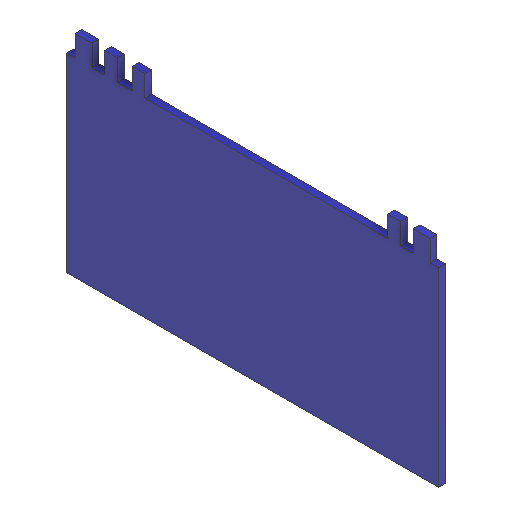
# Autodesk Inventor part: PCB_2
Saved by Autodesk Inventor 2025.2 (Build 292293000, 293)
## iProperties
Created: 2025-03-09
Part Number: PCB_2
Material: Generic
Document SubType Name: Modeling
Designer: ahorat
Density: 1 g/cm^3
Appearance: Default
Author: ahorat
Autodesk Inventor part; units mm, degrees
ref_plane "YZ Plane" through (0, 0, 0) normal (1, 0, 0) x (0, 1, 0)
ref_plane "XZ Plane" through (0, 0, 0) normal (0, 1, 0) x (-1, 0, 0)
ref_plane "XY Plane" through (0, 0, 0) normal (0, 0, 1) x (1, 0, 0)
sketch "Sketch1" plane through (0, 0, 0) normal (0, 0, 1) x (1, 0, 0)
  line L0 (-44, -22.5) -> (44, -22.5)
  line L1 (44, -22.5) -> (44, 22.5)
  line L2 (44, 22.5) -> (-44, 22.5)
  line L3 (-44, 22.5) -> (-44, -22.5)
  line L4 (-44, -22.5) -> (44, 22.5) construction
  line L5 (44, -22.5) -> (-44, 22.5) construction
  line L6 (-42, 22.5) -> (-42, 27.5)
  line L7 (-42, 27.5) -> (-38, 27.5)
  line L8 (-38, 27.5) -> (-38, 22.5)
  line L9 (-35, 22.5) -> (-35, 27.5)
  line L10 (-35, 27.5) -> (-32, 27.5)
  line L11 (-32, 27.5) -> (-32, 22.5)
  line L12 (-28.5, 22.5) -> (-28.5, 27.5)
  line L13 (-28.5, 27.5) -> (-25.5, 27.5)
  line L14 (-25.5, 27.5) -> (-25.5, 22.5)
  line L15 (32, 22.5) -> (32, 27.5)
  line L16 (32, 27.5) -> (35, 27.5)
  line L17 (35, 27.5) -> (35, 22.5)
  line L18 (38, 22.5) -> (38, 27.5)
  line L19 (38, 27.5) -> (42, 27.5)
  line L20 (42, 27.5) -> (42, 22.5)
  point P0 (0, 0)
  point P1 (-28.5, 25)
  point P2 (-40, 27.5)
  dimension "d0" = 45
  dimension "d1" = 88
  dimension "d2" = 4
  dimension "d3" = 3
  dimension "d4" = 3
  dimension "d5" = 3
  dimension "d6" = 4
  dimension "d7" = 2
  dimension "d8" = 3
  dimension "d9" = 3.5
  dimension "d10" = 2
  dimension "d11" = 3
  dimension "d12" = 5
  constraints: 40 end point, 7 point on line, 6 vertical, 5 parallel, 4 midpoint, 3 horizontal, 2 perpendicular, 13 other
  measures "d0" distance of L0.end L1.end
  measures "d1" distance of L1.end L3.start
  measures "d2" distance of L6.end L7.end
  measures "d3" distance of L9.end L10.end
  measures "d4" distance of L12.end L13.end
  measures "d5" distance of L15.end L16.end
  measures "d6" distance of L18.end L19.end
  measures "d7" distance between parallel lines of L6 L3
  measures "d8" distance between parallel lines of L9 L8
  measures "d9" distance from line of point (-28.5, 25) L11
  measures "d10" distance between parallel lines of L20 L1
  measures "d11" distance between parallel lines of L18 L17
extrude "Extrusion1" add sketch "Sketch1" along normal blind 1.6
body "Solid1"
